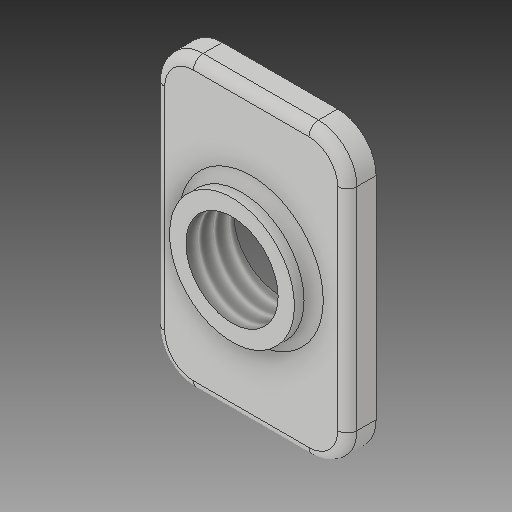
# Autodesk Inventor part: M5 Tee Nut_CPY
Saved by Autodesk Inventor 2018 (Build 220112000, 112)
## iProperties
Created: 2016-07-11
Part Number: M5 Tee Nut_CPY
Material: Generic
Document SubType Name: Modeling
Designer: User
Density: 1 g/cm^3
Appearance: Default
Mass: 0.206466 g
Surface Area: 3.70535 cm^2
Volume: 0.206466 cm^3
Author: joshm
Autodesk Inventor part; units mm, degrees
ref_plane "YZ Plane" through (0, 0, 0) normal (1, 0, 0) x (0, 1, 0)
ref_plane "XZ Plane" through (0, 0, 0) normal (0, 1, 0) x (-1, 0, 0)
ref_plane "XY Plane" through (0, 0, 0) normal (0, 0, 1) x (1, 0, 0)
sketch "Sketch1" plane through (0, 0, 0) normal (0, 0, 1) x (1, 0, 0)
  line L0 (2, 0) -> (8, 0)
  line L1 (10, 2) -> (10, 13)
  line L2 (8, 15) -> (2, 15)
  line L3 (0, 13) -> (0, 2)
  circle A0 centre (5, 7.5) radius 2.4
  arc A1 (10, 13) -> (8, 15) centre (8, 13) ccw
  arc A2 (2, 15) -> (0, 13) centre (2, 13) ccw
  arc A3 (0, 2) -> (2, 0) centre (2, 2) ccw
  arc A4 (8, 0) -> (10, 2) centre (8, 2) ccw
  point P0 (0, 0)
  point P1 (10, 15)
  point P2 (10, 0)
  point P3 (0, 15)
  dimension "d0" = 10
  dimension "d1" = 15
  dimension "d2" = 4.8
  dimension "d3" = 2
  constraints: 8 end point, 8 point on circle, 8 point on line, 8 tangent, 5 centre point, 3 equal radius, 2 parallel, 1 horizontal, 1 perpendicular
  measures "d0" distance of point (0, 15) point (10, 15)
  measures "d1" distance of point (10, 15) point (10, 0)
  measures "d2" diameter of A0
  measures "d3" radius of A1
extrude "Extrusion1" add sketch "Sketch1" along normal blind 1.5
sketch "Sketch2" plane through (0, 0, 1.5) normal (0, 0, 1) x (1, 0, 0)
  circle A0 centre (5, 7.5) radius 2.4 projected
  circle A1 centre (5, 7.5) radius 3.25
  point P0 (0, 0)
  dimension "d6" = 6.5
  constraints: 1 centre point, 1 coincident
  measures "d6" diameter of A1
extrude "Extrusion2" add sketch "Sketch2" along normal blind 1
fillet "Fillet1" radius 0.5 1 edges at (1.75, 7.5, 1.5)
thread "Thread1" size "M5x0.8" class "6H" standard "ANSI Metric M Profile" full length
fillet "Fillet2" radius 0.5 8 edges at (0.5858, 0.5858, 1.5) (5, 0, 1.5) (9.4142, 0.5858, 1.5) (10, 7.5, 1.5) (9.4142, 14.4142, 1.5) (5, 15, 1.5) (0.5858, 14.4142, 1.5) (0, 7.5, 1.5)
body "Solid1"
